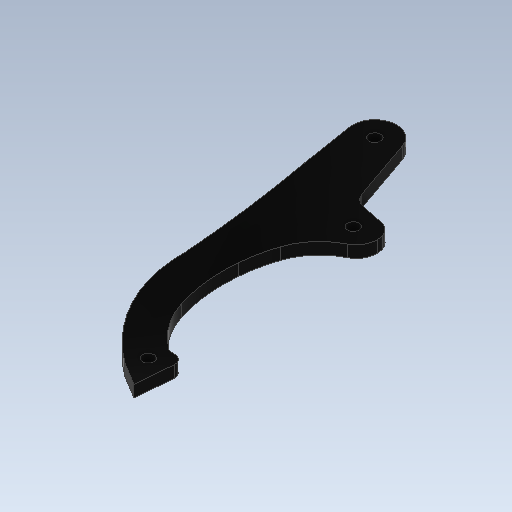
# Autodesk Inventor part: claw2
Saved by Autodesk Inventor 2020.3 (Build 243373000, 373)
## iProperties
Created: 2017-02-15
Part Number: claw2
Material: ABS Plastic
Document SubType Name: Modeling
Designer: Nanjar
Density: 1.06 g/cm^3
Appearance: Smooth - White
Mass: 3.4578 g
Surface Area: 29.075 cm^2
Volume: 3.26208 cm^3
Author: Nanjar
Autodesk Inventor part; units mm, degrees
ref_plane "YZ Plane" through (0, 0, 0) normal (1, 0, 0) x (0, 1, 0)
ref_plane "XZ Plane" through (0, 0, 0) normal (0, 1, 0) x (-1, 0, 0)
ref_plane "XY Plane" through (0, 0, 0) normal (0, 0, 1) x (1, 0, 0)
sketch "Sketch4" plane through (0, 0, 0) normal (0, 1, 0) x (-1, 0, 0)
  arc A0 (8.5248, -5.2299) -> (8.4715, -3.5145) centre (2.5627, -4.5564) ccw
  circle A1 centre (-13.8365, 17.7403) radius 1.5
  circle A2 centre (2.9812, -4.5435) radius 1.5
  arc A3 (-18.1395, 21.8135) -> (-18.0355, 13.56) centre (-13.8365, 17.7403) ccw
  arc A4 (-9.0304, 31.4366) -> (-7.2225, 40.1949) centre (-45.2058, 43.4695) ccw
  arc A5 (-18.1395, 21.8135) -> (-9.0304, 31.4366) centre (-23.8893, 36.3791) ccw
  line L0 (6.3335, 9.9302) -> (8.4977, -3.6654)
  circle A6 centre (-16.5155, 72.4101) radius 3.2
  line L1 (-20.6719, 80.2448) -> (-14.7774, 76.6686)
  arc A7 (-2.5338, 62.5638) -> (-14.7774, 76.6686) centre (-39.7178, 42.6529) ccw
  arc A8 (1.8655, 44.4721) -> (-2.5338, 62.5638) centre (-35.3105, 45.0128) ccw
  arc A9 (1.8655, 44.4721) -> (6.3335, 9.9302) centre (325.703, 68.8005) ccw
  line L2 (-21.6848, 68.4625) -> (-20.6719, 80.2448)
  line L3 (-18.8545, 68.4625) -> (-21.6848, 68.4625)
  line L4 (-18.8545, 68.4625) -> (-17.8545, 68.4625)
  arc A10 (-9.0296, 56.61) -> (-17.8545, 68.4625) centre (-31.443, 49.1333) ccw
  arc A11 (-7.2225, 40.1949) -> (-9.0296, 56.61) centre (-48.1916, 43.9919) ccw
  line L5 (-8.5324, 11.672) -> (-2.2983, -6.3679)
  line L6 (-8.5324, 11.672) -> (-18.0355, 13.56)
  arc A12 (8.4977, -3.6654) -> (8.4715, -3.5145) centre (2.9812, -4.5435) ccw
  arc A13 (-2.2983, -6.3679) -> (8.5248, -5.2299) centre (2.9812, -4.5435) ccw
  arc A14 (8.4977, -3.6654) -> (8.4715, -3.5145) centre (2.9812, -4.5435) ccw
  point P0 (0, 0)
  point P1 (-5.4967, 17.4778)
  point P2 (-7.3422, 22.2297)
  point P3 (-8.8923, 40.8853)
  point P4 (7.4044, -1.132)
  point P5 (0, 0)
  dimension "d11" = 3
  dimension "d23" = 6.4
  constraints: 25 point on circle, 15 centre point, 14 end point, 5 tangent, 2 coincident, 2 horizontal
  measures "d11" diameter of A2
  measures "d23" diameter of A6
extrude "Extrusion4" add sketch "Sketch4" along normal blind 3 contours A13 L5 L6 A3 A5 A4 A11 A10 L4 L3 L2 L1 A7 A8 A9 L0 A0 | A6
fillet "Fillet5" radius 5.2 1 edges at (18.1395, 1.5, 21.8135)
fillet "Fillet6" radius 2 1 edges at (17.8545, 1.5, 68.4625)
fillet "Fillet8" radius 2.2 1 edges at (21.6848, 1.5, 68.4625)
sketch "Sketch7" plane through (0, 3, 0) normal (0, 1, 0) x (1, 0, 0)
  circle A0 centre (16.7249, -72.6774) radius 1.5
  dimension "d31" = 3
  constraints: 1 centre point
  measures "d31" diameter of A0
extrude "Extrusion7" cut sketch "Sketch7" against normal through all
fillet "Fillet9" radius 4 1 edges at (18.0355, 1.5, 13.56)
fillet "Fillet10" radius 4 1 edges at (8.5324, 1.5, 11.672)
body "Solid4"
